Autodesk Fusion 360 part; units mm, degrees
(part 4 of 4)
  line L351 (84.3651, -4.7303) -> (80.3652, -4.7299)
  line L352 (80.3652, -4.7299) -> (80.3651, -4.2302)
  spline S234 degree 3 poles (80.3651, -4.2302) (80.3651, -3.9545) (80.1412, -3.7306) (79.8651, -3.7302) knots 0 0 0 0 1 1 1 1
  line L353 (79.8651, -3.7302) -> (75.8651, -3.7302)
  spline S235 degree 3 poles (75.8651, -3.7302) (75.589, -3.7306) (75.3651, -3.9545) (75.3651, -4.2302) knots 0 0 0 0 1 1 1 1
  line L354 (75.3651, -4.2302) -> (75.365, -4.7299)
  line L355 (75.365, -4.7299) -> (71.3651, -4.7303)
  spline S236 degree 3 poles (71.3651, -4.7303) (71.089, -4.7306) (70.8651, -4.9545) (70.8651, -5.2303) knots 0 0 0 0 1 1 1 1
  line L356 (70.8651, -5.2303) -> (70.8651, -18.2311)
  spline S237 degree 3 poles (70.8651, -18.2311) (70.8651, -18.5068) (71.089, -18.7306) (71.3651, -18.7311) knots 0 0 0 0 1 1 1 1
  line L357 (71.3651, -18.7311) -> (75.365, -18.7316)
  line L358 (75.365, -18.7316) -> (75.3651, -19.2312)
  spline S238 degree 3 poles (75.3651, -19.2312) (75.3651, -19.5068) (75.589, -19.7306) (75.8651, -19.7312) knots 0 0 0 0 1 1 1 1
  line L359 (75.8651, -19.7312) -> (79.8651, -19.7312)
  spline S239 degree 3 poles (79.8651, -19.7312) (80.1412, -19.7306) (80.3651, -19.5068) (80.3651, -19.2312) knots 0 0 0 0 1 1 1 1
  spline S240 degree 3 poles (0.1475, -86.7531) (16.4755, -91.7568) (32.7176, -97.0425) (49.0596, -102.0002) knots 0 0 0 0 1 1 1 1
  line L360 (49.0596, -102.0002) -> (83.4763, -102.2808)
  line L361 (83.4763, -102.2808) -> (140.4459, -128.7386)
  line L362 (140.4459, -128.7386) -> (156.2758, -98.5813)
  line L363 (156.2758, -98.5813) -> (146.2984, -77.639)
  line L364 (146.2984, -77.639) -> (146.2614, -1.7872)
  line L365 (146.2614, -1.7872) -> (86.8333, -0.05)
  line L366 (86.8333, -0.05) -> (68.7094, -0.05)
  line L367 (68.7094, -0.05) -> (0.05, -7.7891)
  line L368 (0.05, -7.7891) -> (0.1475, -86.7531)
extrude "Extrude2" [suppressed]
move_body "Move2" [suppressed]
sketch "KeyCutouts" plane through (0, 0, 0) normal (0, 0, 1) x (1, 0, 0)
  arc A0 (71.3766, -18.7315) -> (70.8766, -18.2315) centre (71.3766, -18.2315) cw
  arc A1 (84.8766, -18.2315) -> (84.3766, -18.7315) centre (84.3766, -18.2315) cw
  arc A2 (84.3766, -4.7315) -> (84.8766, -5.2315) centre (84.3766, -5.2315) cw
  arc A3 (70.8766, -5.2315) -> (71.3766, -4.7315) centre (71.3766, -5.2315) cw
  line L0 (71.3766, -18.7315) -> (84.3766, -18.7315)
  line L1 (84.3766, -4.7315) -> (71.3766, -4.7315)
  line L2 (84.8766, -18.2315) -> (84.8766, -5.2315)
  line L3 (70.8766, -5.2315) -> (70.8766, -18.2315)
  arc A4 (52.3266, -21.1128) -> (51.8266, -20.6128) centre (52.3266, -20.6128) cw
  arc A5 (65.8266, -20.6128) -> (65.3266, -21.1128) centre (65.3266, -20.6128) cw
  arc A6 (65.3266, -7.1128) -> (65.8266, -7.6128) centre (65.3266, -7.6128) cw
  arc A7 (51.8266, -7.6128) -> (52.3266, -7.1128) centre (52.3266, -7.6128) cw
  line L4 (52.3266, -21.1128) -> (65.3266, -21.1128)
  line L5 (65.3266, -7.1128) -> (52.3266, -7.1128)
  line L6 (65.8266, -20.6128) -> (65.8266, -7.6128)
  line L7 (51.8266, -7.6128) -> (51.8266, -20.6128)
  arc A8 (90.4266, -21.1128) -> (89.9266, -20.6128) centre (90.4266, -20.6128) cw
  arc A9 (103.9266, -20.6128) -> (103.4266, -21.1128) centre (103.4266, -20.6128) cw
  arc A10 (103.4266, -7.1128) -> (103.9266, -7.6128) centre (103.4266, -7.6128) cw
  arc A11 (89.9266, -7.6128) -> (90.4266, -7.1128) centre (90.4266, -7.6128) cw
  line L8 (90.4266, -21.1128) -> (103.4266, -21.1128)
  line L9 (103.4266, -7.1128) -> (90.4266, -7.1128)
  line L10 (103.9266, -20.6128) -> (103.9266, -7.6128)
  line L11 (89.9266, -7.6128) -> (89.9266, -20.6128)
  arc A12 (109.4766, -23.494) -> (108.9766, -22.994) centre (109.4766, -22.994) cw
  arc A13 (122.9766, -22.994) -> (122.4766, -23.494) centre (122.4766, -22.994) cw
  arc A14 (122.4766, -9.494) -> (122.9766, -9.994) centre (122.4766, -9.994) cw
  arc A15 (108.9766, -9.994) -> (109.4766, -9.494) centre (109.4766, -9.994) cw
  line L12 (109.4766, -23.494) -> (122.4766, -23.494)
  line L13 (122.4766, -9.494) -> (109.4766, -9.494)
  line L14 (122.9766, -22.994) -> (122.9766, -9.994)
  line L15 (108.9766, -9.994) -> (108.9766, -22.994)
  arc A16 (9.4641, -25.8753) -> (8.9641, -25.3753) centre (9.4641, -25.3753) cw
  arc A17 (22.9641, -25.3753) -> (22.4641, -25.8753) centre (22.4641, -25.3753) cw
  arc A18 (22.4641, -11.8753) -> (22.9641, -12.3753) centre (22.4641, -12.3753) cw
  arc A19 (8.9641, -12.3753) -> (9.4641, -11.8753) centre (9.4641, -12.3753) cw
  line L16 (9.4641, -25.8753) -> (22.4641, -25.8753)
  line L17 (22.4641, -11.8753) -> (9.4641, -11.8753)
  line L18 (22.9641, -25.3753) -> (22.9641, -12.3753)
  line L19 (8.9641, -12.3753) -> (8.9641, -25.3753)
  arc A20 (33.2766, -25.8753) -> (32.7766, -25.3753) centre (33.2766, -25.3753) cw
  arc A21 (46.7766, -25.3753) -> (46.2766, -25.8753) centre (46.2766, -25.3753) cw
  arc A22 (46.2766, -11.8753) -> (46.7766, -12.3753) centre (46.2766, -12.3753) cw
  arc A23 (32.7766, -12.3753) -> (33.2766, -11.8753) centre (33.2766, -12.3753) cw
  line L20 (33.2766, -25.8753) -> (46.2766, -25.8753)
  line L21 (46.2766, -11.8753) -> (33.2766, -11.8753)
  line L22 (46.7766, -25.3753) -> (46.7766, -12.3753)
  line L23 (32.7766, -12.3753) -> (32.7766, -25.3753)
  arc A24 (71.3766, -37.7815) -> (70.8766, -37.2815) centre (71.3766, -37.2815) cw
  arc A25 (84.8766, -37.2815) -> (84.3766, -37.7815) centre (84.3766, -37.2815) cw
  arc A26 (84.3766, -23.7815) -> (84.8766, -24.2815) centre (84.3766, -24.2815) cw
  arc A27 (70.8766, -24.2815) -> (71.3766, -23.7815) centre (71.3766, -24.2815) cw
  line L24 (71.3766, -37.7815) -> (84.3766, -37.7815)
  line L25 (84.3766, -23.7815) -> (71.3766, -23.7815)
  line L26 (84.8766, -37.2815) -> (84.8766, -24.2815)
  line L27 (70.8766, -24.2815) -> (70.8766, -37.2815)
  arc A28 (52.3266, -40.1628) -> (51.8266, -39.6628) centre (52.3266, -39.6628) cw
  arc A29 (65.8266, -39.6628) -> (65.3266, -40.1628) centre (65.3266, -39.6628) cw
  arc A30 (65.3266, -26.1628) -> (65.8266, -26.6628) centre (65.3266, -26.6628) cw
  arc A31 (51.8266, -26.6628) -> (52.3266, -26.1628) centre (52.3266, -26.6628) cw
  line L28 (52.3266, -40.1628) -> (65.3266, -40.1628)
  line L29 (65.3266, -26.1628) -> (52.3266, -26.1628)
  line L30 (65.8266, -39.6628) -> (65.8266, -26.6628)
  line L31 (51.8266, -26.6628) -> (51.8266, -39.6628)
  arc A32 (90.4266, -40.1628) -> (89.9266, -39.6628) centre (90.4266, -39.6628) cw
  arc A33 (103.9266, -39.6628) -> (103.4266, -40.1628) centre (103.4266, -39.6628) cw
  arc A34 (103.4266, -26.1628) -> (103.9266, -26.6628) centre (103.4266, -26.6628) cw
  arc A35 (89.9266, -26.6628) -> (90.4266, -26.1628) centre (90.4266, -26.6628) cw
  line L32 (90.4266, -40.1628) -> (103.4266, -40.1628)
  line L33 (103.4266, -26.1628) -> (90.4266, -26.1628)
  line L34 (103.9266, -39.6628) -> (103.9266, -26.6628)
  line L35 (89.9266, -26.6628) -> (89.9266, -39.6628)
  arc A36 (109.4766, -42.544) -> (108.9766, -42.044) centre (109.4766, -42.044) cw
  arc A37 (122.9766, -42.044) -> (122.4766, -42.544) centre (122.4766, -42.044) cw
  arc A38 (122.4766, -28.544) -> (122.9766, -29.044) centre (122.4766, -29.044) cw
  arc A39 (108.9766, -29.044) -> (109.4766, -28.544) centre (109.4766, -29.044) cw
  line L36 (109.4766, -42.544) -> (122.4766, -42.544)
  line L37 (122.4766, -28.544) -> (109.4766, -28.544)
  line L38 (122.9766, -42.044) -> (122.9766, -29.044)
  line L39 (108.9766, -29.044) -> (108.9766, -42.044)
  arc A40 (9.4641, -44.9253) -> (8.9641, -44.4253) centre (9.4641, -44.4253) cw
  arc A41 (22.9641, -44.4253) -> (22.4641, -44.9253) centre (22.4641, -44.4253) cw
  arc A42 (22.4641, -30.9253) -> (22.9641, -31.4253) centre (22.4641, -31.4253) cw
  arc A43 (8.9641, -31.4253) -> (9.4641, -30.9253) centre (9.4641, -31.4253) cw
  line L40 (9.4641, -44.9253) -> (22.4641, -44.9253)
  line L41 (22.4641, -30.9253) -> (9.4641, -30.9253)
  line L42 (22.9641, -44.4253) -> (22.9641, -31.4253)
  line L43 (8.9641, -31.4253) -> (8.9641, -44.4253)
  arc A44 (33.2766, -44.9253) -> (32.7766, -44.4253) centre (33.2766, -44.4253) cw
  arc A45 (46.7766, -44.4253) -> (46.2766, -44.9253) centre (46.2766, -44.4253) cw
  arc A46 (46.2766, -30.9253) -> (46.7766, -31.4253) centre (46.2766, -31.4253) cw
  arc A47 (32.7766, -31.4253) -> (33.2766, -30.9253) centre (33.2766, -31.4253) cw
  line L44 (33.2766, -44.9253) -> (46.2766, -44.9253)
  line L45 (46.2766, -30.9253) -> (33.2766, -30.9253)
  line L46 (46.7766, -44.4253) -> (46.7766, -31.4253)
  line L47 (32.7766, -31.4253) -> (32.7766, -44.4253)
  arc A48 (71.3766, -56.8315) -> (70.8766, -56.3315) centre (71.3766, -56.3315) cw
  arc A49 (84.8766, -56.3315) -> (84.3766, -56.8315) centre (84.3766, -56.3315) cw
  arc A50 (84.3766, -42.8315) -> (84.8766, -43.3315) centre (84.3766, -43.3315) cw
  arc A51 (70.8766, -43.3315) -> (71.3766, -42.8315) centre (71.3766, -43.3315) cw
  line L48 (71.3766, -56.8315) -> (84.3766, -56.8315)
  line L49 (84.3766, -42.8315) -> (71.3766, -42.8315)
  line L50 (84.8766, -56.3315) -> (84.8766, -43.3315)
  line L51 (70.8766, -43.3315) -> (70.8766, -56.3315)
  arc A52 (52.3266, -59.2128) -> (51.8266, -58.7128) centre (52.3266, -58.7128) cw
  arc A53 (65.8266, -58.7128) -> (65.3266, -59.2128) centre (65.3266, -58.7128) cw
  arc A54 (65.3266, -45.2128) -> (65.8266, -45.7128) centre (65.3266, -45.7128) cw
  arc A55 (51.8266, -45.7128) -> (52.3266, -45.2128) centre (52.3266, -45.7128) cw
  line L52 (52.3266, -59.2128) -> (65.3266, -59.2128)
  line L53 (65.3266, -45.2128) -> (52.3266, -45.2128)
  line L54 (65.8266, -58.7128) -> (65.8266, -45.7128)
  line L55 (51.8266, -45.7128) -> (51.8266, -58.7128)
  arc A56 (90.4266, -59.2128) -> (89.9266, -58.7128) centre (90.4266, -58.7128) cw
  arc A57 (103.9266, -58.7128) -> (103.4266, -59.2128) centre (103.4266, -58.7128) cw
  arc A58 (103.4266, -45.2128) -> (103.9266, -45.7128) centre (103.4266, -45.7128) cw
  arc A59 (89.9266, -45.7128) -> (90.4266, -45.2128) centre (90.4266, -45.7128) cw
  line L56 (90.4266, -59.2128) -> (103.4266, -59.2128)
  line L57 (103.4266, -45.2128) -> (90.4266, -45.2128)
  line L58 (103.9266, -58.7128) -> (103.9266, -45.7128)
  line L59 (89.9266, -45.7128) -> (89.9266, -58.7128)
  arc A60 (109.4766, -61.594) -> (108.9766, -61.094) centre (109.4766, -61.094) cw
  arc A61 (122.9766, -61.094) -> (122.4766, -61.594) centre (122.4766, -61.094) cw
  arc A62 (122.4766, -47.594) -> (122.9766, -48.094) centre (122.4766, -48.094) cw
  arc A63 (108.9766, -48.094) -> (109.4766, -47.594) centre (109.4766, -48.094) cw
  line L60 (109.4766, -61.594) -> (122.4766, -61.594)
  line L61 (122.4766, -47.594) -> (109.4766, -47.594)
  line L62 (122.9766, -61.094) -> (122.9766, -48.094)
  line L63 (108.9766, -48.094) -> (108.9766, -61.094)
  arc A64 (9.4641, -63.9753) -> (8.9641, -63.4753) centre (9.4641, -63.4753) cw
  arc A65 (22.9641, -63.4753) -> (22.4641, -63.9753) centre (22.4641, -63.4753) cw
  arc A66 (22.4641, -49.9753) -> (22.9641, -50.4753) centre (22.4641, -50.4753) cw
  arc A67 (8.9641, -50.4753) -> (9.4641, -49.9753) centre (9.4641, -50.4753) cw
  line L64 (9.4641, -63.9753) -> (22.4641, -63.9753)
  line L65 (22.4641, -49.9753) -> (9.4641, -49.9753)
  line L66 (22.9641, -63.4753) -> (22.9641, -50.4753)
  line L67 (8.9641, -50.4753) -> (8.9641, -63.4753)
  arc A68 (33.2766, -63.9753) -> (32.7766, -63.4753) centre (33.2766, -63.4753) cw
  arc A69 (46.7766, -63.4753) -> (46.2766, -63.9753) centre (46.2766, -63.4753) cw
  arc A70 (46.2766, -49.9753) -> (46.7766, -50.4753) centre (46.2766, -50.4753) cw
  arc A71 (32.7766, -50.4753) -> (33.2766, -49.9753) centre (33.2766, -50.4753) cw
  line L68 (33.2766, -63.9753) -> (46.2766, -63.9753)
  line L69 (46.2766, -49.9753) -> (33.2766, -49.9753)
  line L70 (46.7766, -63.4753) -> (46.7766, -50.4753)
  line L71 (32.7766, -50.4753) -> (32.7766, -63.4753)
  arc A72 (128.5266, -71.119) -> (128.0266, -70.619) centre (128.5266, -70.619) cw
  arc A73 (142.0266, -70.619) -> (141.5266, -71.119) centre (141.5266, -70.619) cw
  arc A74 (141.5266, -57.119) -> (142.0266, -57.619) centre (141.5266, -57.619) cw
  arc A75 (128.0266, -57.619) -> (128.5266, -57.119) centre (128.5266, -57.619) cw
  line L72 (128.5266, -71.119) -> (141.5266, -71.119)
  line L73 (141.5266, -57.119) -> (128.5266, -57.119)
  line L74 (142.0266, -70.619) -> (142.0266, -57.619)
  line L75 (128.0266, -57.619) -> (128.0266, -70.619)
  arc A76 (71.3766, -75.8815) -> (70.8766, -75.3815) centre (71.3766, -75.3815) cw
  arc A77 (84.8766, -75.3815) -> (84.3766, -75.8815) centre (84.3766, -75.3815) cw
  arc A78 (84.3766, -61.8815) -> (84.8766, -62.3815) centre (84.3766, -62.3815) cw
  arc A79 (70.8766, -62.3815) -> (71.3766, -61.8815) centre (71.3766, -62.3815) cw
  line L76 (71.3766, -75.8815) -> (84.3766, -75.8815)
  line L77 (84.3766, -61.8815) -> (71.3766, -61.8815)
  line L78 (84.8766, -75.3815) -> (84.8766, -62.3815)
  line L79 (70.8766, -62.3815) -> (70.8766, -75.3815)
  arc A80 (52.3266, -78.2628) -> (51.8266, -77.7628) centre (52.3266, -77.7628) cw
  arc A81 (65.8266, -77.7628) -> (65.3266, -78.2628) centre (65.3266, -77.7628) cw
  arc A82 (65.3266, -64.2628) -> (65.8266, -64.7628) centre (65.3266, -64.7628) cw
  arc A83 (51.8266, -64.7628) -> (52.3266, -64.2628) centre (52.3266, -64.7628) cw
  line L80 (52.3266, -78.2628) -> (65.3266, -78.2628)
  line L81 (65.3266, -64.2628) -> (52.3266, -64.2628)
  line L82 (65.8266, -77.7628) -> (65.8266, -64.7628)
  line L83 (51.8266, -64.7628) -> (51.8266, -77.7628)
  arc A84 (90.4266, -78.2628) -> (89.9266, -77.7628) centre (90.4266, -77.7628) cw
  arc A85 (103.9266, -77.7628) -> (103.4266, -78.2628) centre (103.4266, -77.7628) cw
  arc A86 (103.4266, -64.2628) -> (103.9266, -64.7628) centre (103.4266, -64.7628) cw
  arc A87 (89.9266, -64.7628) -> (90.4266, -64.2628) centre (90.4266, -64.7628) cw
  line L84 (90.4266, -78.2628) -> (103.4266, -78.2628)
  line L85 (103.4266, -64.2628) -> (90.4266, -64.2628)
  line L86 (103.9266, -77.7628) -> (103.9266, -64.7628)
  line L87 (89.9266, -64.7628) -> (89.9266, -77.7628)
  arc A88 (109.4766, -80.644) -> (108.9766, -80.144) centre (109.4766, -80.144) cw
  arc A89 (122.9766, -80.144) -> (122.4766, -80.644) centre (122.4766, -80.144) cw
  arc A90 (122.4766, -66.644) -> (122.9766, -67.144) centre (122.4766, -67.144) cw
  arc A91 (108.9766, -67.144) -> (109.4766, -66.644) centre (109.4766, -67.144) cw
  line L88 (109.4766, -80.644) -> (122.4766, -80.644)
  line L89 (122.4766, -66.644) -> (109.4766, -66.644)
  line L90 (122.9766, -80.144) -> (122.9766, -67.144)
  line L91 (108.9766, -67.144) -> (108.9766, -80.144)
  arc A92 (9.4641, -83.0253) -> (8.9641, -82.5253) centre (9.4641, -82.5253) cw
  arc A93 (22.9641, -82.5253) -> (22.4641, -83.0253) centre (22.4641, -82.5253) cw
  arc A94 (22.4641, -69.0253) -> (22.9641, -69.5253) centre (22.4641, -69.5253) cw
  arc A95 (8.9641, -69.5253) -> (9.4641, -69.0253) centre (9.4641, -69.5253) cw
  line L92 (9.4641, -83.0253) -> (22.4641, -83.0253)
  line L93 (22.4641, -69.0253) -> (9.4641, -69.0253)
  line L94 (22.9641, -82.5253) -> (22.9641, -69.5253)
  line L95 (8.9641, -69.5253) -> (8.9641, -82.5253)
  arc A96 (33.2766, -83.0253) -> (32.7766, -82.5253) centre (33.2766, -82.5253) cw
  arc A97 (46.7766, -82.5253) -> (46.2766, -83.0253) centre (46.2766, -82.5253) cw
  arc A98 (46.2766, -69.0253) -> (46.7766, -69.5253) centre (46.2766, -69.5253) cw
  arc A99 (32.7766, -69.5253) -> (33.2766, -69.0253) centre (33.2766, -69.5253) cw
  line L96 (33.2766, -83.0253) -> (46.2766, -83.0253)
  line L97 (46.2766, -69.0253) -> (33.2766, -69.0253)
  line L98 (46.7766, -82.5253) -> (46.7766, -69.5253)
  line L99 (32.7766, -69.5253) -> (32.7766, -82.5253)
  arc A100 (71.3766, -94.9315) -> (70.8766, -94.4315) centre (71.3766, -94.4315) cw
  arc A101 (84.8766, -94.4315) -> (84.3766, -94.9315) centre (84.3766, -94.4315) cw
  arc A102 (84.3766, -80.9315) -> (84.8766, -81.4315) centre (84.3766, -81.4315) cw
  arc A103 (70.8766, -81.4315) -> (71.3766, -80.9315) centre (71.3766, -81.4315) cw
  line L100 (71.3766, -94.9315) -> (84.3766, -94.9315)
  line L101 (84.3766, -80.9315) -> (71.3766, -80.9315)
  line L102 (84.8766, -94.4315) -> (84.8766, -81.4315)
  line L103 (70.8766, -81.4315) -> (70.8766, -94.4315)
  arc A104 (52.3266, -97.3128) -> (51.8266, -96.8128) centre (52.3266, -96.8128) cw
  arc A105 (65.8266, -96.8128) -> (65.3266, -97.3128) centre (65.3266, -96.8128) cw
  arc A106 (65.3266, -83.3128) -> (65.8266, -83.8128) centre (65.3266, -83.8128) cw
  arc A107 (51.8266, -83.8128) -> (52.3266, -83.3128) centre (52.3266, -83.8128) cw
  line L104 (52.3266, -97.3128) -> (65.3266, -97.3128)
  line L105 (65.3266, -83.3128) -> (52.3266, -83.3128)
  line L106 (65.8266, -96.8128) -> (65.8266, -83.8128)
  line L107 (51.8266, -83.8128) -> (51.8266, -96.8128)
  arc A108 (90.4266, -97.3128) -> (89.9266, -96.8128) centre (90.4266, -96.8128) cw
  arc A109 (103.9266, -96.8128) -> (103.4266, -97.3128) centre (103.4266, -96.8128) cw
  arc A110 (103.4266, -83.3128) -> (103.9266, -83.8128) centre (103.4266, -83.8128) cw
  arc A111 (89.9266, -83.8128) -> (90.4266, -83.3128) centre (90.4266, -83.8128) cw
  line L108 (90.4266, -97.3128) -> (103.4266, -97.3128)
  line L109 (103.4266, -83.3128) -> (90.4266, -83.3128)
  line L110 (103.9266, -96.8128) -> (103.9266, -83.8128)
  line L111 (89.9266, -83.8128) -> (89.9266, -96.8128)
  line L112 (147.9205, -103.841) -> (136.3376, -97.9382)
  spline S0 degree 3 poles (136.3376, -97.9382) (136.0915, -97.8128) (135.7904, -97.9107) (135.665, -98.1572) knots 0 0 0 0 1 1 1 1
  line L113 (135.665, -98.1572) -> (129.7632, -109.7392)
  spline S1 degree 3 poles (129.7632, -109.7392) (129.6378, -109.9858) (129.7356, -110.2869) (129.9817, -110.4128) knots 0 0 0 0 1 1 1 1
  line L114 (129.9817, -110.4128) -> (141.5647, -116.3138)
  spline S2 degree 3 poles (141.5647, -116.3138) (141.8108, -116.4395) (142.1119, -116.3417) (142.2373, -116.0957) knots 0 0 0 0 1 1 1 1
  line L115 (142.2373, -116.0957) -> (148.1391, -104.5128)
  spline S3 degree 3 poles (148.1391, -104.5128) (148.2645, -104.2665) (148.1667, -103.9654) (147.9205, -103.841) knots 0 0 0 0 1 1 1 1
  line L116 (122.261, -110.1937) -> (128.1627, -98.6102)
  spline S4 degree 3 poles (128.1627, -98.6102) (128.2881, -98.3641) (128.1903, -98.063) (127.9442, -97.9379) knots 0 0 0 0 1 1 1 1
  line L117 (127.9442, -97.9379) -> (116.3612, -92.0355)
  spline S5 degree 3 poles (116.3612, -92.0355) (116.1151, -91.9104) (115.814, -92.0082) (115.6887, -92.2546) knots 0 0 0 0 1 1 1 1
  line L118 (115.6887, -92.2546) -> (109.7868, -103.8379)
  spline S6 degree 3 poles (109.7868, -103.8379) (109.6614, -104.0834) (109.7592, -104.3845) (110.0052, -104.5101) knots 0 0 0 0 1 1 1 1
  line L119 (110.0052, -104.5101) -> (121.5884, -110.4112)
  spline S7 degree 3 poles (121.5884, -110.4112) (121.8344, -110.5371) (122.1355, -110.4393) (122.261, -110.1937) knots 0 0 0 0 1 1 1 1
  spline S8 degree 3 poles (0.1475, -86.7531) (16.4755, -91.7568) (32.7176, -97.0425) (49.0596, -102.0002) knots 0 0 0 0 1 1 1 1
  line L120 (49.0596, -102.0002) -> (83.4763, -102.2808)
  line L121 (83.4763, -102.2808) -> (140.4459, -128.7386)
  line L122 (140.4459, -128.7386) -> (156.2758, -98.5813)
  line L123 (156.2758, -98.5813) -> (146.2984, -77.639)
  line L124 (146.2984, -77.639) -> (146.2614, -1.7872)
  line L125 (146.2614, -1.7872) -> (86.8333, -0.05)
  line L126 (86.8333, -0.05) -> (68.7094, -0.05)
  line L127 (68.7094, -0.05) -> (0.05, -7.7891)
  line L128 (0.05, -7.7891) -> (0.1475, -86.7531)
extrude "Extrude3" [suppressed]
sketch "KeyPlate" plane through (0, 0, 0) normal (0, 0, 1) x (1, 0, 0)
  arc A0 (71.3766, -18.7315) -> (70.8766, -18.2315) centre (71.3766, -18.2315) cw
  arc A1 (84.8766, -18.2315) -> (84.3766, -18.7315) centre (84.3766, -18.2315) cw
  arc A2 (84.3766, -4.7315) -> (84.8766, -5.2315) centre (84.3766, -5.2315) cw
  arc A3 (70.8766, -5.2315) -> (71.3766, -4.7315) centre (71.3766, -5.2315) cw
  line L0 (71.3766, -18.7315) -> (84.3766, -18.7315)
  line L1 (84.3766, -4.7315) -> (71.3766, -4.7315)
  line L2 (84.8766, -18.2315) -> (84.8766, -5.2315)
  line L3 (70.8766, -5.2315) -> (70.8766, -18.2315)
  arc A4 (52.3266, -21.1128) -> (51.8266, -20.6128) centre (52.3266, -20.6128) cw
  arc A5 (65.8266, -20.6128) -> (65.3266, -21.1128) centre (65.3266, -20.6128) cw
  arc A6 (65.3266, -7.1128) -> (65.8266, -7.6128) centre (65.3266, -7.6128) cw
  arc A7 (51.8266, -7.6128) -> (52.3266, -7.1128) centre (52.3266, -7.6128) cw
  line L4 (52.3266, -21.1128) -> (65.3266, -21.1128)
  line L5 (65.3266, -7.1128) -> (52.3266, -7.1128)
  line L6 (65.8266, -20.6128) -> (65.8266, -7.6128)
  line L7 (51.8266, -7.6128) -> (51.8266, -20.6128)
  arc A8 (90.4266, -21.1128) -> (89.9266, -20.6128) centre (90.4266, -20.6128) cw
  arc A9 (103.9266, -20.6128) -> (103.4266, -21.1128) centre (103.4266, -20.6128) cw
  arc A10 (103.4266, -7.1128) -> (103.9266, -7.6128) centre (103.4266, -7.6128) cw
  arc A11 (89.9266, -7.6128) -> (90.4266, -7.1128) centre (90.4266, -7.6128) cw
  line L8 (90.4266, -21.1128) -> (103.4266, -21.1128)
  line L9 (103.4266, -7.1128) -> (90.4266, -7.1128)
  line L10 (103.9266, -20.6128) -> (103.9266, -7.6128)
  line L11 (89.9266, -7.6128) -> (89.9266, -20.6128)
  arc A12 (109.4766, -23.494) -> (108.9766, -22.994) centre (109.4766, -22.994) cw
  arc A13 (122.9766, -22.994) -> (122.4766, -23.494) centre (122.4766, -22.994) cw
  arc A14 (122.4766, -9.494) -> (122.9766, -9.994) centre (122.4766, -9.994) cw
  arc A15 (108.9766, -9.994) -> (109.4766, -9.494) centre (109.4766, -9.994) cw
  line L12 (109.4766, -23.494) -> (122.4766, -23.494)
  line L13 (122.4766, -9.494) -> (109.4766, -9.494)
  line L14 (122.9766, -22.994) -> (122.9766, -9.994)
  line L15 (108.9766, -9.994) -> (108.9766, -22.994)
  arc A16 (9.4641, -25.8753) -> (8.9641, -25.3753) centre (9.4641, -25.3753) cw
  arc A17 (22.9641, -25.3753) -> (22.4641, -25.8753) centre (22.4641, -25.3753) cw
  arc A18 (22.4641, -11.8753) -> (22.9641, -12.3753) centre (22.4641, -12.3753) cw
  arc A19 (8.9641, -12.3753) -> (9.4641, -11.8753) centre (9.4641, -12.3753) cw
  line L16 (9.4641, -25.8753) -> (22.4641, -25.8753)
  line L17 (22.4641, -11.8753) -> (9.4641, -11.8753)
  line L18 (22.9641, -25.3753) -> (22.9641, -12.3753)
  line L19 (8.9641, -12.3753) -> (8.9641, -25.3753)
  arc A20 (33.2766, -25.8753) -> (32.7766, -25.3753) centre (33.2766, -25.3753) cw
  arc A21 (46.7766, -25.3753) -> (46.2766, -25.8753) centre (46.2766, -25.3753) cw
  arc A22 (46.2766, -11.8753) -> (46.7766, -12.3753) centre (46.2766, -12.3753) cw
  arc A23 (32.7766, -12.3753) -> (33.2766, -11.8753) centre (33.2766, -12.3753) cw
  line L20 (33.2766, -25.8753) -> (46.2766, -25.8753)
  line L21 (46.2766, -11.8753) -> (33.2766, -11.8753)
  line L22 (46.7766, -25.3753) -> (46.7766, -12.3753)
  line L23 (32.7766, -12.3753) -> (32.7766, -25.3753)
  arc A24 (71.3766, -37.7815) -> (70.8766, -37.2815) centre (71.3766, -37.2815) cw
  arc A25 (84.8766, -37.2815) -> (84.3766, -37.7815) centre (84.3766, -37.2815) cw
  arc A26 (84.3766, -23.7815) -> (84.8766, -24.2815) centre (84.3766, -24.2815) cw
  arc A27 (70.8766, -24.2815) -> (71.3766, -23.7815) centre (71.3766, -24.2815) cw
  line L24 (71.3766, -37.7815) -> (84.3766, -37.7815)
  line L25 (84.3766, -23.7815) -> (71.3766, -23.7815)
  line L26 (84.8766, -37.2815) -> (84.8766, -24.2815)
  line L27 (70.8766, -24.2815) -> (70.8766, -37.2815)
  arc A28 (52.3266, -40.1628) -> (51.8266, -39.6628) centre (52.3266, -39.6628) cw
  arc A29 (65.8266, -39.6628) -> (65.3266, -40.1628) centre (65.3266, -39.6628) cw
  arc A30 (65.3266, -26.1628) -> (65.8266, -26.6628) centre (65.3266, -26.6628) cw
  arc A31 (51.8266, -26.6628) -> (52.3266, -26.1628) centre (52.3266, -26.6628) cw
  line L28 (52.3266, -40.1628) -> (65.3266, -40.1628)
  line L29 (65.3266, -26.1628) -> (52.3266, -26.1628)
  line L30 (65.8266, -39.6628) -> (65.8266, -26.6628)
  line L31 (51.8266, -26.6628) -> (51.8266, -39.6628)
  arc A32 (90.4266, -40.1628) -> (89.9266, -39.6628) centre (90.4266, -39.6628) cw
  arc A33 (103.9266, -39.6628) -> (103.4266, -40.1628) centre (103.4266, -39.6628) cw
  arc A34 (103.4266, -26.1628) -> (103.9266, -26.6628) centre (103.4266, -26.6628) cw
  arc A35 (89.9266, -26.6628) -> (90.4266, -26.1628) centre (90.4266, -26.6628) cw
  line L32 (90.4266, -40.1628) -> (103.4266, -40.1628)
  line L33 (103.4266, -26.1628) -> (90.4266, -26.1628)
  line L34 (103.9266, -39.6628) -> (103.9266, -26.6628)
  line L35 (89.9266, -26.6628) -> (89.9266, -39.6628)
  arc A36 (109.4766, -42.544) -> (108.9766, -42.044) centre (109.4766, -42.044) cw
  arc A37 (122.9766, -42.044) -> (122.4766, -42.544) centre (122.4766, -42.044) cw
  arc A38 (122.4766, -28.544) -> (122.9766, -29.044) centre (122.4766, -29.044) cw
  arc A39 (108.9766, -29.044) -> (109.4766, -28.544) centre (109.4766, -29.044) cw
  line L36 (109.4766, -42.544) -> (122.4766, -42.544)
  line L37 (122.4766, -28.544) -> (109.4766, -28.544)
  line L38 (122.9766, -42.044) -> (122.9766, -29.044)
  line L39 (108.9766, -29.044) -> (108.9766, -42.044)
  arc A40 (9.4641, -44.9253) -> (8.9641, -44.4253) centre (9.4641, -44.4253) cw
  arc A41 (22.9641, -44.4253) -> (22.4641, -44.9253) centre (22.4641, -44.4253) cw
  arc A42 (22.4641, -30.9253) -> (22.9641, -31.4253) centre (22.4641, -31.4253) cw
  arc A43 (8.9641, -31.4253) -> (9.4641, -30.9253) centre (9.4641, -31.4253) cw
  line L40 (9.4641, -44.9253) -> (22.4641, -44.9253)
  line L41 (22.4641, -30.9253) -> (9.4641, -30.9253)
  line L42 (22.9641, -44.4253) -> (22.9641, -31.4253)
  line L43 (8.9641, -31.4253) -> (8.9641, -44.4253)
  arc A44 (33.2766, -44.9253) -> (32.7766, -44.4253) centre (33.2766, -44.4253) cw
  arc A45 (46.7766, -44.4253) -> (46.2766, -44.9253) centre (46.2766, -44.4253) cw
  arc A46 (46.2766, -30.9253) -> (46.7766, -31.4253) centre (46.2766, -31.4253) cw
  arc A47 (32.7766, -31.4253) -> (33.2766, -30.9253) centre (33.2766, -31.4253) cw
  line L44 (33.2766, -44.9253) -> (46.2766, -44.9253)
  line L45 (46.2766, -30.9253) -> (33.2766, -30.9253)
  line L46 (46.7766, -44.4253) -> (46.7766, -31.4253)
  line L47 (32.7766, -31.4253) -> (32.7766, -44.4253)
  arc A48 (71.3766, -56.8315) -> (70.8766, -56.3315) centre (71.3766, -56.3315) cw
  arc A49 (84.8766, -56.3315) -> (84.3766, -56.8315) centre (84.3766, -56.3315) cw
  arc A50 (84.3766, -42.8315) -> (84.8766, -43.3315) centre (84.3766, -43.3315) cw
  arc A51 (70.8766, -43.3315) -> (71.3766, -42.8315) centre (71.3766, -43.3315) cw
  line L48 (71.3766, -56.8315) -> (84.3766, -56.8315)
  line L49 (84.3766, -42.8315) -> (71.3766, -42.8315)
  line L50 (84.8766, -56.3315) -> (84.8766, -43.3315)
  line L51 (70.8766, -43.3315) -> (70.8766, -56.3315)
  arc A52 (52.3266, -59.2128) -> (51.8266, -58.7128) centre (52.3266, -58.7128) cw
  arc A53 (65.8266, -58.7128) -> (65.3266, -59.2128) centre (65.3266, -58.7128) cw
  arc A54 (65.3266, -45.2128) -> (65.8266, -45.7128) centre (65.3266, -45.7128) cw
  arc A55 (51.8266, -45.7128) -> (52.3266, -45.2128) centre (52.3266, -45.7128) cw
  line L52 (52.3266, -59.2128) -> (65.3266, -59.2128)
  line L53 (65.3266, -45.2128) -> (52.3266, -45.2128)
  line L54 (65.8266, -58.7128) -> (65.8266, -45.7128)
  line L55 (51.8266, -45.7128) -> (51.8266, -58.7128)
  arc A56 (90.4266, -59.2128) -> (89.9266, -58.7128) centre (90.4266, -58.7128) cw
  arc A57 (103.9266, -58.7128) -> (103.4266, -59.2128) centre (103.4266, -58.7128) cw
  arc A58 (103.4266, -45.2128) -> (103.9266, -45.7128) centre (103.4266, -45.7128) cw
  arc A59 (89.9266, -45.7128) -> (90.4266, -45.2128) centre (90.4266, -45.7128) cw
  line L56 (90.4266, -59.2128) -> (103.4266, -59.2128)
  line L57 (103.4266, -45.2128) -> (90.4266, -45.2128)
  line L58 (103.9266, -58.7128) -> (103.9266, -45.7128)
  line L59 (89.9266, -45.7128) -> (89.9266, -58.7128)
  arc A60 (109.4766, -61.594) -> (108.9766, -61.094) centre (109.4766, -61.094) cw
  arc A61 (122.9766, -61.094) -> (122.4766, -61.594) centre (122.4766, -61.094) cw
  arc A62 (122.4766, -47.594) -> (122.9766, -48.094) centre (122.4766, -48.094) cw
  arc A63 (108.9766, -48.094) -> (109.4766, -47.594) centre (109.4766, -48.094) cw
  line L60 (109.4766, -61.594) -> (122.4766, -61.594)
  line L61 (122.4766, -47.594) -> (109.4766, -47.594)
  line L62 (122.9766, -61.094) -> (122.9766, -48.094)
  line L63 (108.9766, -48.094) -> (108.9766, -61.094)
  arc A64 (9.4641, -63.9753) -> (8.9641, -63.4753) centre (9.4641, -63.4753) cw
  arc A65 (22.9641, -63.4753) -> (22.4641, -63.9753) centre (22.4641, -63.4753) cw
  arc A66 (22.4641, -49.9753) -> (22.9641, -50.4753) centre (22.4641, -50.4753) cw
  arc A67 (8.9641, -50.4753) -> (9.4641, -49.9753) centre (9.4641, -50.4753) cw
  line L64 (9.4641, -63.9753) -> (22.4641, -63.9753)
  line L65 (22.4641, -49.9753) -> (9.4641, -49.9753)
  line L66 (22.9641, -63.4753) -> (22.9641, -50.4753)
  line L67 (8.9641, -50.4753) -> (8.9641, -63.4753)
  arc A68 (33.2766, -63.9753) -> (32.7766, -63.4753) centre (33.2766, -63.4753) cw
  arc A69 (46.7766, -63.4753) -> (46.2766, -63.9753) centre (46.2766, -63.4753) cw
  arc A70 (46.2766, -49.9753) -> (46.7766, -50.4753) centre (46.2766, -50.4753) cw
  arc A71 (32.7766, -50.4753) -> (33.2766, -49.9753) centre (33.2766, -50.4753) cw
  line L68 (33.2766, -63.9753) -> (46.2766, -63.9753)
  line L69 (46.2766, -49.9753) -> (33.2766, -49.9753)
  line L70 (46.7766, -63.4753) -> (46.7766, -50.4753)
  line L71 (32.7766, -50.4753) -> (32.7766, -63.4753)
  arc A72 (128.5266, -71.119) -> (128.0266, -70.619) centre (128.5266, -70.619) cw
  arc A73 (142.0266, -70.619) -> (141.5266, -71.119) centre (141.5266, -70.619) cw
  arc A74 (141.5266, -57.119) -> (142.0266, -57.619) centre (141.5266, -57.619) cw
  arc A75 (128.0266, -57.619) -> (128.5266, -57.119) centre (128.5266, -57.619) cw
  line L72 (128.5266, -71.119) -> (141.5266, -71.119)
  line L73 (141.5266, -57.119) -> (128.5266, -57.119)
  line L74 (142.0266, -70.619) -> (142.0266, -57.619)
  line L75 (128.0266, -57.619) -> (128.0266, -70.619)
  arc A76 (71.3766, -75.8815) -> (70.8766, -75.3815) centre (71.3766, -75.3815) cw
  arc A77 (84.8766, -75.3815) -> (84.3766, -75.8815) centre (84.3766, -75.3815) cw
  arc A78 (84.3766, -61.8815) -> (84.8766, -62.3815) centre (84.3766, -62.3815) cw
  arc A79 (70.8766, -62.3815) -> (71.3766, -61.8815) centre (71.3766, -62.3815) cw
  line L76 (71.3766, -75.8815) -> (84.3766, -75.8815)
  line L77 (84.3766, -61.8815) -> (71.3766, -61.8815)
  line L78 (84.8766, -75.3815) -> (84.8766, -62.3815)
  line L79 (70.8766, -62.3815) -> (70.8766, -75.3815)
  arc A80 (52.3266, -78.2628) -> (51.8266, -77.7628) centre (52.3266, -77.7628) cw
  arc A81 (65.8266, -77.7628) -> (65.3266, -78.2628) centre (65.3266, -77.7628) cw
  arc A82 (65.3266, -64.2628) -> (65.8266, -64.7628) centre (65.3266, -64.7628) cw
  arc A83 (51.8266, -64.7628) -> (52.3266, -64.2628) centre (52.3266, -64.7628) cw
  line L80 (52.3266, -78.2628) -> (65.3266, -78.2628)
  line L81 (65.3266, -64.2628) -> (52.3266, -64.2628)
  line L82 (65.8266, -77.7628) -> (65.8266, -64.7628)
  line L83 (51.8266, -64.7628) -> (51.8266, -77.7628)
  arc A84 (90.4266, -78.2628) -> (89.9266, -77.7628) centre (90.4266, -77.7628) cw
  arc A85 (103.9266, -77.7628) -> (103.4266, -78.2628) centre (103.4266, -77.7628) cw
  arc A86 (103.4266, -64.2628) -> (103.9266, -64.7628) centre (103.4266, -64.7628) cw
  arc A87 (89.9266, -64.7628) -> (90.4266, -64.2628) centre (90.4266, -64.7628) cw
  line L84 (90.4266, -78.2628) -> (103.4266, -78.2628)
  line L85 (103.4266, -64.2628) -> (90.4266, -64.2628)
  line L86 (103.9266, -77.7628) -> (103.9266, -64.7628)
  line L87 (89.9266, -64.7628) -> (89.9266, -77.7628)
  arc A88 (109.4766, -80.644) -> (108.9766, -80.144) centre (109.4766, -80.144) cw
  arc A89 (122.9766, -80.144) -> (122.4766, -80.644) centre (122.4766, -80.144) cw
  arc A90 (122.4766, -66.644) -> (122.9766, -67.144) centre (122.4766, -67.144) cw
  arc A91 (108.9766, -67.144) -> (109.4766, -66.644) centre (109.4766, -67.144) cw
  line L88 (109.4766, -80.644) -> (122.4766, -80.644)
  line L89 (122.4766, -66.644) -> (109.4766, -66.644)
  line L90 (122.9766, -80.144) -> (122.9766, -67.144)
  line L91 (108.9766, -67.144) -> (108.9766, -80.144)
  arc A92 (9.4641, -83.0253) -> (8.9641, -82.5253) centre (9.4641, -82.5253) cw
  arc A93 (22.9641, -82.5253) -> (22.4641, -83.0253) centre (22.4641, -82.5253) cw
  arc A94 (22.4641, -69.0253) -> (22.9641, -69.5253) centre (22.4641, -69.5253) cw
  arc A95 (8.9641, -69.5253) -> (9.4641, -69.0253) centre (9.4641, -69.5253) cw
  line L92 (9.4641, -83.0253) -> (22.4641, -83.0253)
  line L93 (22.4641, -69.0253) -> (9.4641, -69.0253)
  line L94 (22.9641, -82.5253) -> (22.9641, -69.5253)
  line L95 (8.9641, -69.5253) -> (8.9641, -82.5253)
  arc A96 (33.2766, -83.0253) -> (32.7766, -82.5253) centre (33.2766, -82.5253) cw
  arc A97 (46.7766, -82.5253) -> (46.2766, -83.0253) centre (46.2766, -82.5253) cw
  arc A98 (46.2766, -69.0253) -> (46.7766, -69.5253) centre (46.2766, -69.5253) cw
  arc A99 (32.7766, -69.5253) -> (33.2766, -69.0253) centre (33.2766, -69.5253) cw
  line L96 (33.2766, -83.0253) -> (46.2766, -83.0253)
  line L97 (46.2766, -69.0253) -> (33.2766, -69.0253)
  line L98 (46.7766, -82.5253) -> (46.7766, -69.5253)
  line L99 (32.7766, -69.5253) -> (32.7766, -82.5253)
  arc A100 (71.3766, -94.9315) -> (70.8766, -94.4315) centre (71.3766, -94.4315) cw
  arc A101 (84.8766, -94.4315) -> (84.3766, -94.9315) centre (84.3766, -94.4315) cw
  arc A102 (84.3766, -80.9315) -> (84.8766, -81.4315) centre (84.3766, -81.4315) cw
  arc A103 (70.8766, -81.4315) -> (71.3766, -80.9315) centre (71.3766, -81.4315) cw
  line L100 (71.3766, -94.9315) -> (84.3766, -94.9315)
  line L101 (84.3766, -80.9315) -> (71.3766, -80.9315)
  line L102 (84.8766, -94.4315) -> (84.8766, -81.4315)
  line L103 (70.8766, -81.4315) -> (70.8766, -94.4315)
  arc A104 (52.3266, -97.3128) -> (51.8266, -96.8128) centre (52.3266, -96.8128) cw
  arc A105 (65.8266, -96.8128) -> (65.3266, -97.3128) centre (65.3266, -96.8128) cw
  arc A106 (65.3266, -83.3128) -> (65.8266, -83.8128) centre (65.3266, -83.8128) cw
  arc A107 (51.8266, -83.8128) -> (52.3266, -83.3128) centre (52.3266, -83.8128) cw
  line L104 (52.3266, -97.3128) -> (65.3266, -97.3128)
  line L105 (65.3266, -83.3128) -> (52.3266, -83.3128)
  line L106 (65.8266, -96.8128) -> (65.8266, -83.8128)
  line L107 (51.8266, -83.8128) -> (51.8266, -96.8128)
  arc A108 (90.4266, -97.3128) -> (89.9266, -96.8128) centre (90.4266, -96.8128) cw
  arc A109 (103.9266, -96.8128) -> (103.4266, -97.3128) centre (103.4266, -96.8128) cw
  arc A110 (103.4266, -83.3128) -> (103.9266, -83.8128) centre (103.4266, -83.8128) cw
  arc A111 (89.9266, -83.8128) -> (90.4266, -83.3128) centre (90.4266, -83.8128) cw
  line L108 (90.4266, -97.3128) -> (103.4266, -97.3128)
  line L109 (103.4266, -83.3128) -> (90.4266, -83.3128)
  line L110 (103.9266, -96.8128) -> (103.9266, -83.8128)
  line L111 (89.9266, -83.8128) -> (89.9266, -96.8128)
  arc A112 (129.9817, -110.4123) -> (129.7632, -109.7398) centre (130.2087, -109.9668) cw
  arc A113 (142.2373, -116.0957) -> (141.5648, -116.3142) centre (141.7918, -115.8687) cw
  arc A114 (147.9206, -103.8401) -> (148.1392, -104.5126) centre (147.6936, -104.2856) cw
  arc A115 (135.665, -98.1567) -> (136.3375, -97.9382) centre (136.1105, -98.3837) cw
  line L112 (129.9817, -110.4123) -> (141.5648, -116.3142)
  line L113 (147.9206, -103.8401) -> (136.3375, -97.9382)
  line L114 (142.2373, -116.0957) -> (148.1392, -104.5126)
  line L115 (135.665, -98.1578) -> (129.7632, -109.7386)
  arc A116 (110.0053, -104.5099) -> (109.7868, -103.8374) centre (110.2323, -104.0644) cw
  arc A117 (122.2609, -110.1932) -> (121.5884, -110.4118) centre (121.8154, -109.9663) cw
  arc A118 (127.9442, -97.9377) -> (128.1627, -98.6102) centre (127.7172, -98.3832) cw
  arc A119 (115.6886, -92.2543) -> (116.3611, -92.0358) centre (116.1342, -92.4813) cw
  line L116 (110.0053, -104.5099) -> (121.5884, -110.4106)
  line L117 (127.9442, -97.9377) -> (116.3611, -92.0358)
  line L118 (122.2609, -110.1932) -> (128.1627, -98.6102)
  line L119 (115.6886, -92.2543) -> (109.7868, -103.8374)
  spline S0 degree 3 poles (0.1475, -86.7531) (16.4755, -91.7568) (32.7176, -97.0425) (49.0596, -102.0002) knots 0 0 0 0 1 1 1 1
  line L120 (49.0596, -102.0002) -> (83.4763, -102.2808)
  line L121 (83.4763, -102.2808) -> (140.4459, -128.7386)
  line L122 (140.4459, -128.7386) -> (156.2758, -98.5813)
  line L123 (156.2758, -98.5813) -> (146.2984, -77.639)
  line L124 (146.2984, -77.639) -> (146.2614, -1.7872)
  line L125 (146.2614, -1.7872) -> (86.8333, -0.05)
  line L126 (86.8333, -0.05) -> (68.7094, -0.05)
  line L127 (68.7094, -0.05) -> (0.05, -7.7891)
  line L128 (0.05, -7.7891) -> (0.1475, -86.7531)
extrude "Extrude1" [suppressed]
move_body "Move1" [suppressed]
hidden bodies 2
named bodies: "SupportPlate", "KeyCutouts", "lh keplate", "rh plate"
